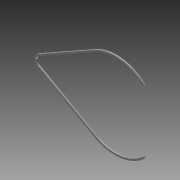
# Autodesk Inventor part: neck chain 1.1
Saved by Autodesk Inventor 2011 SP1 (Build 150282100, 282)
## iProperties
Created: 2012-01-20
Part Number: neck chain 1.1
Document SubType Name: Modeling
Designer: Christopher
Density: 1 g/cm^3
Author: Christopher
Autodesk Inventor part; units mm, degrees
ref_plane "YZ Plane" through (0, 0, 0) normal (1, 0, 0) x (0, 1, 0)
ref_plane "XZ Plane" through (0, 0, 0) normal (0, 1, 0) x (-1, 0, 0)
ref_plane "XY Plane" through (0, 0, 0) normal (0, 0, 1) x (1, 0, 0)
sketch "Sketch1" plane through (0, 0, 0) normal (0, 0, 1) x (1, 0, 0)
  circle A0 centre (0, 0) radius 162.56
  circle A1 centre (-292.1, 0) radius 19.05
  line L0 (-301.4593, 16.5923) -> (-79.8664, 141.5878)
  line L1 (-301.4593, -16.5923) -> (-79.8664, -141.5878)
  line L2 (-305.4851, -21.6121) -> (-91.0253, -142.5839)
  line L3 (-304.6003, 22.1112) -> (-91.0253, 142.5839)
  arc A2 (-304.6003, 22.1112) -> (-305.4851, -21.6121) centre (-292.1212, -0.0119) ccw
  arc A3 (114.1664, 124.8271) -> (-91.0253, 142.5839) centre (0, 0) ccw
  line L4 (0, 0) -> (114.1664, 124.8271) construction
  line L5 (0, 0) -> (-91.0253, 142.5839) construction
  arc A4 (-91.0253, -142.5839) -> (114.1664, -124.8271) centre (0, 0) ccw
  line L6 (0, 0) -> (114.1664, -124.8271) construction
  line L7 (0, 0) -> (-91.0253, -142.5839) construction
  line L8 (114.1664, -124.8271) -> (109.7108, -119.9554)
  line L9 (114.1664, 124.8271) -> (109.7108, 119.9554)
  arc A5 (109.7108, 119.9554) -> (-87.4728, 137.0192) centre (0, 0) ccw
  line L10 (0, 0) -> (-87.4728, 137.0192) construction
  line L11 (0, 0) -> (109.7108, 119.9554) construction
  arc A6 (-79.8664, -141.5878) -> (116.0924, -113.7907) centre (0, 0) ccw
  line L12 (0, 0) -> (116.0924, -113.7907) construction
  line L13 (0, 0) -> (-79.8664, -141.5878) construction
  dimension "d0" = 325.12
  dimension "d1" = 38.1
  dimension "d2" = 292.1
  dimension "d3" = 6.35
  dimension "d4" = 6.35
  dimension "d5" = 75
  dimension "d6" = 75
  dimension "d7" = 75
  dimension "d8" = 75
  constraints: 28 end point, 16 point on circle, 7 centre point, 6 coincident, 5 tangent, 2 parallel, 2 point on line, 1 horizontal alignment
  measures "d0" diameter of A0
  measures "d1" diameter of A1
  measures "d2" distance of A0.centre A1.centre
  measures "d3" distance between parallel lines of L3 L0
  measures "d4" distance between parallel lines of L2 L1
  measures "d5" angle of L4 L5
  measures "d6" angle of L7 L6
  measures "d7" angle of L11 L10
  measures "d8" angle of L13 L12
extrude "Extrusion1" add sketch "Sketch1" against normal blind 6.35 contours A0 L0 A1 L1 L8 A4 L2 A2 L3 A3 L9
body "Solid1"
